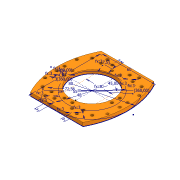
# Autodesk Inventor part: payload-plateV2
Saved by Autodesk Inventor 2020.3 (Build 243373000, 373)
## iProperties
Created: 2021-06-12
Part Number: payload-plateV2
Material: Generic
Document SubType Name: Modeling
Designer: Yusuf
Mass: 15.6692 g
Surface Area: 107.982 cm^2
Volume: 15.6692 cm^3
Density: 1 g/cm^3
Appearance: Orange
Author: Yusuf
Autodesk Inventor part; units mm, degrees
ref_plane "YZ Plane" through (0, 0, 0) normal (1, 0, 0) x (0, 1, 0)
ref_plane "XZ Plane" through (0, 0, 0) normal (0, 1, 0) x (-1, 0, 0)
ref_plane "XY Plane" through (0, 0, 0) normal (0, 0, 1) x (1, 0, 0)
sketch "Sketch1" plane through (0, 0, 0) normal (0, 1, 0) x (-1, 0, 0)
  line L0 (0, 0) -> (60, 0)
  line L1 (60, 0) -> (60, -81)
  line L2 (60, -81) -> (0, -81)
  line L3 (0, -81) -> (0, 0)
  line L4 (45, -21.6284) -> (15, -21.6284) construction
  line L5 (45, -81) -> (45, 0) construction
  line L6 (15, 0) -> (15, -81) construction
  circle A0 centre (40, -73.5) radius 1.5
  circle A1 centre (40, -7.5) radius 1.5
  circle A2 centre (20, -7.5) radius 1.5
  circle A3 centre (20, -73.5) radius 1.5
  line L7 (60, -40.5) -> (0, -40.5) construction
  line L8 (30, 0) -> (30, -81) construction
  circle A4 centre (30, -40.5) radius 24
  circle A5 centre (30, -40.5) radius 27.5
  circle A6 centre (57.1293, -36) radius 1.5
  circle A7 centre (57.1293, -45) radius 1.5
  circle A8 centre (25.5, -13.3707) radius 1.5
  circle A9 centre (34.5, -13.3707) radius 1.5
  circle A10 centre (2.8707, -45) radius 1.5
  circle A11 centre (2.8707, -36) radius 1.5
  circle A12 centre (34.5, -67.6293) radius 1.5
  circle A13 centre (25.5, -67.6293) radius 1.5
  circle A14 centre (30, -40.5) radius 40 construction
  arc A15 (60, -81) -> (60, 0) centre (-17.0125, -40.5) ccw
  circle A16 centre (30, -40.5) radius 36.28 construction
  circle A17 centre (65.9998, -36) radius 1.5
  circle A18 centre (65.9998, -45) radius 1.5
  circle A19 centre (-5.9998, -45) radius 1.5
  circle A20 centre (-5.9998, -36) radius 1.5
  arc A21 (0, 0) -> (0, -81) centre (77.0125, -40.5) ccw
  line L9 (30, -40.5) -> (-3.3536, -73.8536) construction
  circle A22 centre (1.7157, -68.7843) radius 1.5
  circle A23 centre (11.8404, -76.1403) radius 1.5
  circle A24 centre (23.7426, -80.0075) radius 1.5
  circle A25 centre (36.2574, -80.0075) radius 1.5
  circle A26 centre (48.1596, -76.1403) radius 1.5
  circle A27 centre (58.2843, -68.7843) radius 1.5
  circle A28 centre (65.6403, -58.6596) radius 1.5
  circle A29 centre (69.5075, -46.7574) radius 1.5
  circle A30 centre (69.5075, -34.2426) radius 1.5
  circle A31 centre (65.6403, -22.3404) radius 1.5
  circle A32 centre (58.2843, -12.2157) radius 1.5
  circle A33 centre (48.1596, -4.8597) radius 1.5
  circle A34 centre (36.2574, -0.9925) radius 1.5
  circle A35 centre (23.7426, -0.9925) radius 1.5
  circle A36 centre (11.8404, -4.8597) radius 1.5
  circle A37 centre (1.7157, -12.2157) radius 1.5
  circle A38 centre (-5.6403, -22.3404) radius 1.5
  circle A39 centre (-9.5075, -34.2426) radius 1.5
  circle A40 centre (-9.5075, -46.7574) radius 1.5
  circle A41 centre (-5.6403, -58.6596) radius 1.5
  circle A42 centre (48.1596, -68.7843) radius 1.5
  circle A43 centre (48.1596, -12.2157) radius 1.5
  circle A44 centre (11.8404, -12.2157) radius 1.5
  circle A45 centre (11.8404, -68.7843) radius 1.5
  point P0 (30, -21.6284)
  dimension "d31" = 80
  dimension "width" = 60
  dimension "d1" = 81
  dimension "fixed" = 3
  dimension "d6" = 7.5
  dimension "d7" = 5
  dimension "d8" = 30
  dimension "d9" = 3
  dimension "d10" = 7.5
  dimension "d11" = 5
  dimension "d12" = 3
  dimension "d13" = 3
  dimension "d14" = 5
  dimension "d19" = 48
  dimension "d20" = 55
  dimension "d21" = 3
  dimension "d22" = 4.5
  dimension "d23" = 3
  dimension "d24" = 4.5
  dimension "d27" = 360
  dimension "d32" = 72.56
  dimension "d33" = 3
  dimension "d34" = 3
  dimension "d37" = 360
  dimension "d39" = 45
  dimension "d40" = 3
  dimension "d43" = 360
  dimension "d47" = 3
  dimension "d48" = 3
  dimension "d49" = 3
  dimension "d50" = 3
  constraints: 45 centre point, 20 end point, 9 point on circle, 7 horizontal alignment, 7 midpoint, 7 point on line, 5 vertical alignment, 4 coincident, 3 perpendicular, 2 horizontal, 2 parallel, 1 symmetric about line, 72 other
  measures "width" distance of L1.end L2.end
  measures "d1" distance of L0.end L1.end
  measures "fixed" diameter of A0
  measures "d6" distance from line of A0.centre L2
  measures "d7" distance from line of L5 A0.centre
  measures "d8" distance between parallel lines of L6 L5
  measures "d9" diameter of A1
  measures "d10" distance from line of L0 A1.centre
  measures "d11" distance from line of L5 A1.centre
  measures "d12" diameter of A2
  measures "d13" diameter of A3
  measures "d14" distance from line of L6 A2.centre
  measures "d19" diameter of A4
  measures "d20" diameter of A5
  measures "d21" diameter of A6
  measures "d22" distance from line of A6.centre L7
  measures "d23" diameter of A7
  measures "d24" distance from line of L7 A7.centre
  measures "d32" diameter of A16
  measures "d33" diameter of A17
  measures "d34" diameter of A18
  measures "d39" angle of L8 L9
  measures "d40" diameter of A22
  measures "d47" diameter of A42
  measures "d48" diameter of A43
  measures "d49" diameter of A44
  measures "d50" diameter of A45
extrude "Extrusion1" add sketch "Sketch1" along normal blind 4 contours L0 A35 A34 L1 L2 A25 A24 L3 | L3 A21 A40 A39 | L0 A35 | A39 A21 | A24 L2 | A21 A40 | L0 A34 | A25 L2 | A15 A30 A29 L1 | A15 A30 | A29 A15 | A4 | A5 A7 A12 A13 A10 A11 A8 A9 A6 | A6 A5 | A5 A6 | A7 A5 | A5 A7 | A9 A5 | A5 A9 | A12 A5 | A5 A12 | A8 A5 | A5 A8 | A13 A5 | A5 A13 | A11 A5 | A5 A11 | A10 A5 | A5 A10 | A22 | A23 | A26 | A27 | A28 | A31 | A32 | A33 | A36 | A37 | A38 | A41 | A42 | A43 | A44 | A45 picked at (23.6828, -0.8272) picked at (-9.1838, -34.2299) picked at (24.0268, -80.2578) picked at (-9.1838, -46.7701) picked at (35.7864, -0.994) picked at (35.8837, -79.4355) picked at (69.1851, -34.2659) picked at (69.1851, -46.7341)
extrude "Extrusion2" cut sketch "Sketch1" along normal blind 10 contours A4 | A6 A5 | A5 A6 | A7 A5 | A5 A7 | A9 A5 | A5 A9 | A12 A5 | A5 A12 | A8 A5 | A5 A8 | A13 A5 | A5 A13 | A11 A5 | A5 A11 | A10 A5 | A5 A10
extrude "Extrusion3" cut sketch "Sketch1" along normal blind 10 contours A22 | A23 | A26 | A27 | A28 | A31 | A32 | A33 | A36 | A37 | A38 | A41 | A42 | A43 | A44 | A45
equation "\"d8\" = 0.5 * width"
equation "\"d9\" = fixed"
equation "\"d12\" = fixed"
equation "\"d13\" = fixed"
equation "\"d23\" = fixed"
equation "\"d33\" = fixed"
equation "\"d34\" = fixed"
equation "\"d40\" = fixed"
equation "\"d47\" = fixed"
equation "\"d48\" = fixed"
equation "\"d49\" = fixed"
equation "\"d50\" = fixed"
body "Solid1"
